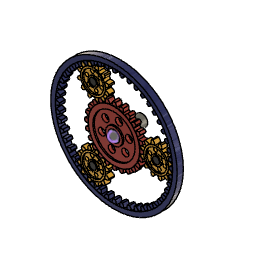
Planetary gearv9 (Autodesk Fusion 360 design; units mm, degrees)
Autodesk Fusion 360 part; units mm, degrees
sketch "Sketch1" plane through (0, 0, 0) normal (0, 0, 1) x (1, 0, 0)
sketch "Sketch2" plane through (0, 0, 0) normal (0, 1, 0) x (1, 0, 0)
  line L0 (91.5, 0) -> (105, 0)
  arc A0 (91.169274, -7.772611) -> (91.169274, 7.772611) centre (0, 0) ccw
  arc A1 (104.938761, -3.585578) -> (104.938761, 3.585578) centre (0, 0) ccw
  line L1 (91.5, 0) -> (105, 0)
  arc A2 (104.895157, -4.69107) -> (104.895157, 4.69107) centre (0, 0) ccw
  arc A3 (93.675267, -7.806683) -> (93.703058, -7.465711) centre (0, 0) ccw
  arc A4 (104.895157, 4.69107) -> (91.152631, 7.965412) centre (90.267606, -26.225164) ccw
  arc A5 (91.152631, -7.965412) -> (104.895157, -4.69107) centre (90.267606, 26.225164) ccw
  arc A6 (91.152631, -7.965412) -> (91.152631, 7.965412) centre (0, 0) ccw
  dimension "d2" = 210
  dimension "d4" = 183
  constraint coincident A0.centre A1.centre
  constraint horizontal L0
  constraint coincident A0 L0.start
  constraint coincident A1 L0.end
  constraint parallel L0 L1
  measures "d2" diameter of A1
  measures "d4" diameter of A0
sketch "Sketch3" plane through (0, 0, 0) normal (0, 1, 0) x (1, 0, 0)
  circle A0 centre (0, 0) radius 91.5
  dimension "d7" = 183
  constraint coincident A0.centre origin
  measures "d7" diameter of A0
extrude "Extrude1" add sketch "Sketch2" along normal mid plane 20 contours L0 A0 A1 L1 A2 A4 A6 | L0 A0 A1 L1 A2 A5 A6 picked at (98.99364, 2.138776) picked at (99.260674, -2.051597) makes body 1
extrude "Extrude2" add sketch "Sketch3" along normal mid plane 22 contours A0 picked at (-10.742379, -25.73436) bodies 1
sketch "Sketch4" plane through (0, -11, 0) normal (0, -1, 0) x (1, 0, 0)
  circle A0 centre (0, 0) radius 91.5
  circle A1 centre (0, 0) radius 20
  circle A2 centre (0, 0) radius 30
  circle A3 centre (0, 0) radius 75
  circle A4 centre (0, 50) radius 12.5
  dimension "d12" = 40
  dimension "d13" = 60
  dimension "d14" = 150
  dimension "d15" = 25
  dimension "d16" = 50
  constraint coincident A0.centre A1.centre
  constraint concentric A1 A3
  measures "d12" diameter of A1
  measures "d13" diameter of A2
  measures "d14" diameter of A3
  measures "d15" diameter of A4
  measures "d16" distance of A0.centre A4.centre
extrude "Extrude3" cut sketch "Sketch4" against normal blind 90 contours A4 picked at (-2.221908, 45.784424) bodies 1
extrude "Extrude4" cut sketch "Sketch4" against normal blind 70 contours A1 picked at (4.742345, -7.111153) bodies 1
extrude "Extrude5" cut sketch "Sketch4" against normal blind 5 contours A3 picked at (-25.803696, 42.802622) bodies 1
pattern_circular "C-Pattern1" count 6 over 360 about axis through (0, -11, 0) along (0, -1, 0) of "Extrude3"
mirror "Mirror1" about plane through (0, 0, 0) normal (0, 1, 0) of "Extrude5"
pattern_circular "C-Pattern2" count 24 over 360 about axis through (0, -11, 0) along (0, -1, 0) of "Extrude1" makes body 2 at (96.17407, 10, 23.555541) makes body 3 at (86.800395, 10, 47.644586) makes body 4 at (71.511417, 10, 68.486732) makes body 5 at (51.349054, 10, 84.661619) makes body 6 at (27.687338, 10, 95.066958) makes body 7 at (2.138776, 10, 98.99364) makes body 8 at (-23.555541, 10, 96.17407) makes body 9 at (-47.644586, 10, 86.800395) makes body 10 at (-68.486732, 10, 71.511417) makes body 11 at (-84.661619, 10, 51.349054) makes body 12 at (-95.066958, 10, 27.687338) makes body 13 at (-98.99364, 10, 2.138776) makes body 14 at (-96.17407, 10, -23.555541) makes body 15 at (-86.800395, 10, -47.644586) makes body 16 at (-71.511417, 10, -68.486732) makes body 17 at (-51.349054, 10, -84.661619) makes body 18 at (-27.687338, 10, -95.066958) makes body 19 at (-2.138776, 10, -98.99364) makes body 20 at (23.555541, 10, -96.17407) makes body 21 at (47.644586, 10, -86.800395) makes body 22 at (68.486732, 10, -71.511417) makes body 23 at (84.661619, 10, -51.349054) makes body 24 at (95.066958, 10, -27.687338)
combine "Combine1" operation add target body 1 tool bodies 5 21 3 4 11 8 2 16 9 10 17 13 18 14 22 15 7 24 20 19 12 23 6
sketch "Sketch5" plane through (0, 0, 0) normal (1, 0, 0) x (0, 1, 0)
sketch "Sketch6" plane through (0, 0, 0) normal (0, 1, 0) x (1, 0, 0)
move_body "Move1" bodies 1 to x (0.99144486, 0, -0.13052619) y (0, 1, 0) z (0.13052619, 0, 0.99144486) at (0, 0, 0)
sketch "Sketch7" plane through (0, -11, 0) normal (0, -1, 0) x (1, 0, 0)
sketch "Sketch8" plane through (0, 0, 0) normal (0, 1, 0) x (-1, 0, 0)
sketch "Sketch9" plane through (0, 0, 0) normal (0, 1, 0) x (1, 0, 0)
  line L0 (92.5, 0) -> (90.367756, 0)
  line L1 (92.5, 0) -> (90.367756, 0)
  arc A0 (92.551232, 2.426745) -> (92.551232, -2.426745) centre (150, 0) ccw
  arc A1 (106.522076, 6.757969) -> (106.522076, -6.757969) centre (150, 0) ccw
  arc A2 (106.522076, 6.757969) -> (92.551232, 2.426745) centre (104.114088, -10.172662) ccw
  line L2 (87.418436, -13.873999) -> (87.171182, -13.928814)
  arc A3 (92.551232, -2.426745) -> (106.522076, -6.757969) centre (104.114088, 10.172662) ccw
  circle A4 centre (150, 0) radius 57.5
  circle A5 centre (150, 0) radius 50
  circle A6 centre (150, 0) radius 47
  circle A7 centre (150, 0) radius 44
  line L3 (150, 0) -> (-12.465908, 21.389043)
  line L4 (150, 0) -> (83.284225, -14.790531)
  line L5 (0, 0) -> (150, 0)
  dimension "d35" = 150
  dimension "d36" = 115
  dimension "d59" = 115
  dimension "d60" = 100
  dimension "d61" = 94
  dimension "d62" = 3
  dimension "d63" = 20
  dimension "d64" = 7.5
  constraint horizontal L0
  constraint coincident A0 L0.start
  constraint concentric A0 A4
  constraint concentric A1 A5
  constraint concentric A4 A6
  constraint concentric A0 A7
  constraint coincident A0.centre A1.centre
  constraint coincident L5.start origin
  constraint horizontal L5
  measures "d35" distance of L5.start A0.centre
  measures "d36" diameter of A0
  measures "d59" diameter of A4
  measures "d60" diameter of A5
  measures "d61" diameter of A6
  measures "d62" distance of A6 A7
  measures "d63" angle of L3 L4
  measures "d64" angle of L3 L5
sketch "Sketch10" plane through (0, 0, 0) normal (0, 1, 0) x (1, 0, 0)
  circle A0 centre (150.006061, -27.515753) radius 6.362097
  circle A1 centre (150, -0.015754) radius 12.5
  circle A2 centre (150, -0.015754) radius 44
  circle A3 centre (173.818728, -13.760505) radius 6.362097
  circle A4 centre (173.812668, 13.739494) radius 6.362097
  circle A5 centre (149.993939, 27.484245) radius 6.362097
  circle A6 centre (126.181272, 13.728997) radius 6.362097
  circle A7 centre (126.187332, -13.771002) radius 6.362097
  dimension "d83" = 25
  dimension "d85" = 88
  dimension "d88" = 360
  dimension "d99" = 27.5
  constraint concentric A1 A2
  measures "d83" diameter of A1
  measures "d85" diameter of A2
extrude "Extrude6" add sketch "Sketch9" along normal mid plane 20 separate body contours A0 A2 A4 A5 L5 | A0 A3 A4 A5 L5 | A5 A6 L3 L5 | A2 A6 L3 | A3 A5 A6 L5 | A1 A2 A6 A7 L3 | A1 A6 A7 L3 L5 | A1 A3 A6 A7 L5 picked at (95.602069, 1.547137) picked at (95.602069, -1.547137) picked at (101.015863, 0.72699) picked at (102.441963, 6.567877) picked at (101.621748, -5.232695) picked at (104.765452, 6.267156) picked at (104.028871, 1.323121) picked at (104.659287, -5.353336) makes body 25
extrude "Extrude7" add sketch "Sketch10" along normal mid plane 22 contours A2 picked at (166.591103, 28.727878) bodies 25
sketch "Sketch11" plane through (0, 11, 0) normal (0, 1, 0) x (-1, 0, 0)
  circle A0 centre (-150.006061, 27.515753) radius 6.362097
  circle A1 centre (-150, 0.015754) radius 44
  circle A2 centre (-126.187332, 13.771002) radius 6.362097
  circle A3 centre (-173.812668, -13.739494) radius 6.362097
  circle A4 centre (-150, 0.015754) radius 12.5
  circle A5 centre (-149.993939, -27.484245) radius 6.362097
  circle A6 centre (-173.818728, 13.760505) radius 6.362097
  circle A7 centre (-126.181272, -13.728997) radius 6.362097
  circle A8 centre (-150, 0.015754) radius 17.5
  circle A9 centre (-150, 0.015754) radius 37.5
  dimension "d89" = 35
  dimension "d90" = 75
  constraint concentric A1 A8
  constraint concentric A8 A9
  measures "d89" diameter of A8
  measures "d90" diameter of A9
extrude "Extrude12" cut sketch "Sketch11" against normal blind 5 contours A9 picked at (-135.039686, 25.934776) bodies 25
mirror "Mirror3" about plane through (0, 0, 0) normal (0, 1, 0) of "Extrude12"
pattern_circular "C-Pattern3" count 12 over 360 about axis through (150, -11, 0.015754) along (0, 1, 0) of "Extrude6"
move_body "Move2" bodies 1 to x (0.99144486, 0, -0.13052619) y (0, 1, 0) z (0.13052619, 0, 0.99144486) at (0, 0, 0)
move_body "Move3" bodies 25 to x (0.96592583, 0, 0.25881905) y (0, 1, 0) z (-0.25881905, 0, 0.96592583) at (5.018691, 0, -38.835026)
pattern_circular "C-Pattern4" count 3 over 360 about axis through (0, -11, 0) along (0, -1, 0) of bodies 25 makes body 26 at (-96.113273, -6, 150.982543) makes body 27 at (-103.856971, -6, -137.563969)
sketch "Sketch12" plane through (0, -11, 0) normal (0, 1, 0) x (-1, 0, 0)
  circle A0 centre (75.309295, -129.725239) radius 12.5
  circle A1 centre (74.690705, 130.082382) radius 12.5
  circle A2 centre (74.690705, 130.082382) radius 12.5
  circle A3 centre (53.335722, -117.411688) radius 6.25
  circle A4 centre (53.335722, -142.411688) radius 6.25
  circle A5 centre (96.636992, -142.411688) radius 6.25
  circle A6 centre (74.986357, -129.911688) radius 12.5
  circle A7 centre (96.636992, -117.411688) radius 6.25
  circle A8 centre (74.986357, -154.911688) radius 6.25
  circle A9 centre (74.986357, -104.911688) radius 6.25
  circle A10 centre (74.986357, -129.911688) radius 44
  circle A11 centre (-150.000002, 0) radius 12.5
  circle A12 centre (-149.903487, 0.003048) radius 12.5
  circle A13 centre (-149.903487, 0.003048) radius 44
  circle A14 centre (-149.903487, 0.003048) radius 37.5
  circle A15 centre (-149.903487, 0.003048) radius 17.5
  circle A16 centre (74.954383, 129.818704) radius 17.5
  circle A17 centre (74.954383, 129.818704) radius 12.5
  circle A18 centre (74.954383, 129.818704) radius 17.5
  circle A19 centre (74.954383, 129.818704) radius 12.5
  dimension "d74" = 25
  dimension "d91" = 25
  constraint concentric A1 A2
  measures "d74" diameter of A1
  measures "d91" diameter of A11
extrude "Extrude9" add sketch "Sketch12" along normal blind 25 separate body contours A0 A6 | A0 A6 | A1 A2 A17 A19 | A1 A2 A17 A19 | A11 A12 picked at (84.794569, -122.005204) picked at (78.862105, -128.065945) picked at (72.090406, 132.999247) picked at (66.043821, 138.729266) picked at (-154.074998, -0.260263) makes body 28 at (-87.747179, 5.666667, -128.480641) makes body 29 at (159.546301, 5.666667, 7.957049) makes body 30 at (-87.12859, 5.666667, 131.32698)
sketch "Sketch13" plane through (0, 0, 0) normal (0, 1, 0) x (1, 0, 0)
  arc A0 (208.586558, -8.258961) -> (208.586558, 8.258961) centre (0, 0) ccw
  arc A1 (194.955329, -4.173691) -> (194.955329, 4.173691) centre (0, 0) ccw
  arc A2 (194.955329, -4.173691) -> (208.586558, -8.258961) centre (225.747486, 73.785652) ccw
  arc A3 (208.586558, 8.258961) -> (194.955329, 4.173691) centre (225.747486, -73.785652) ccw
  dimension "d77" = 390
  dimension "d79" = 417.5
  constraint coincident A0.centre A1.centre
  measures "d77" diameter of A1
  measures "d79" diameter of A0
sketch "Sketch14" plane through (0, 0, 0) normal (0, 1, 0) x (1, 0, 0)
  circle A0 centre (0, 0) radius 208.732775
  circle A1 centre (0, 0) radius 225
  dimension "d92" = 450
  constraint coincident A0.centre A1.centre
  measures "d92" diameter of A1
extrude "Extrude10" add sketch "Sketch13" along normal mid plane 20 separate body contours A0 A1 A2 A3 picked at (202.523574, 0.917875) makes body 31
extrude "Extrude11" add sketch "Sketch14" along normal mid plane 22 separate body contours A1 picked at (217.962779, -21.548172) makes body 32
pattern_circular "C-Pattern5" count 48 over 360 about axis through (0, 11, 0) along (0, -1, 0) of bodies 31 makes body 33 at (207.704622, 3.333333, 20.865098) makes body 34 at (203.204239, 3.333333, 47.797488) makes body 35 at (191.057055, 3.333333, 84.105673) makes body 36 at (180.322106, 3.333333, 105.168915) makes body 37 at (162.778794, 3.333333, 130.689046) makes body 38 at (144.327855, 3.333333, 150.817879) makes body 39 at (127.805938, 3.333333, 165.052127) makes body 40 at (103.579067, 3.333333, 181.240005) makes body 41 at (85.782606, 3.333333, 190.310029) makes body 42 at (54.914576, 3.333333, 201.397497) makes body 43 at (22.690878, 3.333333, 207.5131) makes body 44 at (-4.58914, 3.333333, 208.69955) makes body 45 at (-22.690878, 3.333333, 207.5131) makes body 46 at (-58.448187, 3.333333, 200.400529) makes body 47 at (-73.912049, 3.333333, 195.226974) makes body 48 at (-108.324087, 3.333333, 178.444542) makes body 49 at (-123.407427, 3.333333, 168.366177) makes body 50 at (-150.817879, 3.333333, 144.327855) makes body 51 at (-162.778794, 3.333333, 130.689046) makes body 52 at (-181.240005, 3.333333, 103.579067) makes body 53 at (-194.569431, 3.333333, 75.626048) makes body 54 at (-202.776042, 3.333333, 49.58265) makes body 55 at (-207.5131, 3.333333, 22.690878) makes body 56 at (-208.69955, 3.333333, -4.58914) makes body 57 at (-207.704622, 3.333333, -20.865098) makes body 58 at (-200.400529, 3.333333, -58.448187) makes body 59 at (-195.226974, 3.333333, -73.912049) makes body 60 at (-177.485023, 3.333333, -109.889167) makes body 61 at (-162.778794, 3.333333, -130.689046) makes body 62 at (-144.327855, 3.333333, -150.817879) makes body 63 at (-130.689046, 3.333333, -162.778794) makes body 64 at (-109.889167, 3.333333, -177.485023) makes body 65 at (-75.626048, 3.333333, -194.569431) makes body 66 at (-54.914576, 3.333333, -201.397497) makes body 67 at (-22.690878, 3.333333, -207.5131) makes body 68 at (4.58914, 3.333333, -208.69955) makes body 69 at (20.865098, 3.333333, -207.704622) makes body 70 at (53.141331, 3.333333, -201.872637) makes body 71 at (84.105673, 3.333333, -191.057055) makes body 72 at (109.889167, 3.333333, -177.485023) makes body 73 at (127.805938, 3.333333, -165.052127) makes body 74 at (150.817879, 3.333333, -144.327855) makes body 75 at (162.778794, 3.333333, -130.689046) makes body 76 at (177.485023, 3.333333, -109.889167) makes body 77 at (194.569431, 3.333333, -75.626048) makes body 78 at (202.776042, 3.333333, -49.58265) makes body 79 at (207.5131, 3.333333, -22.690878)
combine "Combine3" operation add target body 32 tool bodies 76 43 34 44 46 66 73 31 58 49 36 55 53 57 60 51 65 75 47 62 41 33 52 48 77 45 37 63 71 50 61 59 40 35 78 74 79 42 64 72 56 39 70 67 38 54 69 68
sketch "Sketch15" plane through (0, -11, 0) normal (0, -1, 0) x (1, 0, 0)
  circle A0 centre (0, 0) radius 30
  circle A1 centre (0, 0) radius 20
  circle A2 centre (0, 0) radius 20
  constraint concentric A0 A2
extrude "Extrude13" add sketch "Sketch15" against normal blind 100 separate body contours A1 A2 picked at (4.742345, -7.111153) makes body 80
sketch "Sketch16" plane through (0, 14, 0) normal (0, 1, 0) x (-1, 0, 0)
  arc A0 (-149.557208, -12.492155) -> (-150.346281, 12.495203) centre (-150.000002, 0) ccw
  arc A1 (-150.346281, 12.495203) -> (-149.557208, -12.492155) centre (-149.903487, 0.003048) ccw
  circle A2 centre (0, 0) radius 20
  line L0 (-150.000002, -20) -> (-45.825757, -20)
  arc A3 (0, -20) -> (0, 20) centre (0, 0) ccw
  line L1 (-45.825757, 20) -> (-150.000002, 20)
  arc A4 (-150.000002, 20) -> (-150.000002, -20) centre (-150.000002, 0) ccw
  line L2 (-150.000002, 0) -> (0, 0) construction
  line L3 (5.59237, -49.68627) -> (57.679493, -139.903813)
  arc A5 (57.679493, -139.903813) -> (92.320509, -119.903813) centre (75.000001, -129.903813) ccw
  line L4 (92.320509, -119.903813) -> (40.233387, -29.68627)
  line L5 (40.233387, 29.68627) -> (92.320509, 119.903813)
  arc A6 (92.320509, 119.903813) -> (57.679493, 139.903813) centre (75.000001, 129.903813) ccw
  line L6 (57.679493, 139.903813) -> (5.59237, 49.68627)
  arc A7 (5.59237, 49.68627) -> (-45.825757, 20) centre (0, 0) ccw
  arc A8 (-45.825757, -20) -> (5.59237, -49.68627) centre (0, 0) ccw
  arc A9 (40.233387, -29.68627) -> (40.233387, 29.68627) centre (0, 0) ccw
  dimension "d106" = 40
  dimension "d107" = 100
  dimension "d108" = 40
  dimension "d110" = 360
  constraint coincident A2.centre A3.centre
  constraint concentric A2 A8
  constraint tangent L0 A3
  constraint tangent A3 L1
  constraint parallel L0 L1
  constraint tangent L1 A4
  constraint tangent L0 A4
  constraint horizontal L2
  constraint concentric A7 A8
  constraint concentric A8 A9
  measures "d106" diameter of A2
  measures "d107" diameter of A8
  measures "d108" diameter of A3
extrude "Extrude14" add sketch "Sketch16" along normal blind 5 separate body contours A0 A1 | L0 L1 A4 L3 A5 L4 L5 A6 L6 A7 A8 A9 picked at (-154.078858, -0.439572) picked at (51.864124, -103.164632) makes body 81
combine "Combine4" operation add target body 81 tool bodies 30 28 29
copy_body "Body->Comp1" bodies 1 removing the originals makes body 82 in component "Component"
copy_body "Body->Comp2" bodies 25 removing the originals makes body 83 in component "Component'"
copy_body "Body->Comp3" bodies 26 removing the originals makes body 84 in component "Component''"
copy_body "Body->Comp4" bodies 27 removing the originals makes body 85 in component "Component'''"
copy_body "Body->Comp5" bodies 32 removing the originals makes body 86 in component "Component''''"
copy_body "Body->Comp6" bodies 80 removing the originals makes body 87 in component "Component'''''"
copy_body "Body->Comp7" bodies 81 removing the originals makes body 88 in component "Component''''''"
component "Component" placed x (1, 0, 0) y (0, 1, 0) z (0, 0, 1) at (0, 0, 0)
component "Component'" placed x (1, 0, 0) y (0, 1, 0) z (0, 0, 1) at (0, 0, 0)
component "Component''" placed x (1, 0, 0) y (0, 1, 0) z (0, 0, 1) at (0, 0, 0)
component "Component'''" placed x (1, 0, 0) y (0, 1, 0) z (0, 0, 1) at (0, 0, 0)
component "Component''''" placed x (1, 0, 0) y (0, 1, 0) z (0, 0, 1) at (0, 0, 0)
component "Component'''''" placed x (1, 0, 0) y (0, 1, 0) z (0, 0, 1) at (0, 0, 0)
component "Component''''''" placed x (1, 0, 0) y (0, 1, 0) z (0, 0, 1) at (0, 0, 0)
equation "d31 = ( 360 / 48 ) * 1 deg"
